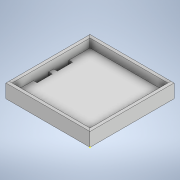
# Autodesk Inventor part: led-compartment
Saved by Autodesk Inventor 2021 (Build 250183000, 183)
## iProperties
Created: 2021-01-17
Part Number: led-compartment
Material: Generic
Document SubType Name: Modeling
Designer: Luke Kamols
Density: 1 g/cm^3
Appearance: Default
Author: Luke Kamols
Autodesk Inventor part; units mm, degrees
ref_plane "YZ Plane" through (0, 0, 0) normal (1, 0, 0) x (0, 1, 0)
ref_plane "XZ Plane" through (0, 0, 0) normal (0, 1, 0) x (-1, 0, 0)
ref_plane "XY Plane" through (0, 0, 0) normal (0, 0, 1) x (1, 0, 0)
sketch "Sketch1" plane through (0, 0, 0) normal (0, 1, 0) x (-1, 0, 0)
  point P0 (0, 0)
sketch "Sketch2" plane through (0, 0, 0) normal (0, 1, 0) x (-1, 0, 0)
  line L0 (0, 0) -> (33.2, 0)
  line L1 (33.2, 0) -> (33.2, -33.2)
  line L2 (33.2, -33.2) -> (0, -33.2)
  line L3 (0, -33.2) -> (0, 0)
  dimension "d0" = 33.2
  dimension "d1" = 33.2
  constraints: 8 end point, 2 parallel, 1 horizontal, 1 perpendicular
  measures "d0" distance of L1.end L2.end
  measures "d1" distance of L0.end L1.end
extrude "Extrusion1" add sketch "Sketch2" along normal blind 2
sketch "Sketch3" plane through (0, 2, 0) normal (0, 1, 0) x (1, 0, 0)
  line L0 (0, 33.2) -> (-33.2, 33.2) projected
  line L1 (-33.2, 33.2) -> (-33.2, 0) projected
  line L2 (-33.2, 0) -> (0, 0) projected
  line L3 (0, 0) -> (0, 33.2) projected
  line L4 (-33.2, 0) -> (0, 0) projected
  line L5 (0, 0) -> (-1.2, 0)
  line L6 (-1.2, 0) -> (-1.2, 1.2)
  line L7 (-1.2, 1.2) -> (-32, 1.2)
  line L8 (-32, 1.2) -> (-32, 32)
  line L9 (-32, 32) -> (-1.2, 32)
  line L10 (-1.2, 32) -> (-1.2, 1.2)
  dimension "d4" = 1.2
  dimension "d5" = 1.2
  dimension "d6" = 30.8
  dimension "d7" = 30.8
  constraints: 12 end point, 2 parallel, 2 perpendicular, 1 horizontal, 1 point on line
  measures "d4" distance of L4.end L5.end
  measures "d5" distance of L5.end L6.end
  measures "d6" distance of L8.end L9.end
  measures "d7" distance of L7.end L8.end
extrude "Extrusion2" add sketch "Sketch3" along normal blind 4
chamfer "Chamfer1" distance 0.6 angle 45 8 edges at (-1.2, 6, -16.6) (-16.6, 6, -32) (-16.6, 6, -33.2) (0, 6, -16.6) (-16.6, 6, 0) (-16.6, 6, -1.2) (-33.2, 6, -16.6) (-32, 6, -16.6)
sketch "Sketch4" plane through (0, 2, 0) normal (0, 1, 0) x (1, 0, 0)
  line L0 (-1.2, 1.2) -> (-1.2, 32) projected
  line L1 (-1.2, 32) -> (-32, 32) projected
  line L2 (-32, 32) -> (-32, 1.2) projected
  line L3 (-32, 1.2) -> (-1.2, 1.2) projected
  line L4 (-1.2, 1.2) -> (-1.2, 32) projected
  line L5 (-1.2, 16.6) -> (-32, 16.6)
  line L6 (-32, 32) -> (-1.2, 32) projected
  line L7 (-16.6, 32) -> (-16.6, 1.2)
  line L8 (-16.6, 16.6) -> (-16.6, 17.6)
  line L9 (-32, 16.6) -> (-32, 17.6)
  line L10 (-32, 1.2) -> (-32, 32) projected
  line L11 (-32, 17.6) -> (-30.5, 17.6)
  line L12 (-30.5, 17.6) -> (-30.5, 23.6)
  line L13 (-30.5, 23.6) -> (-32, 23.6)
  line L14 (-30.5, 16.6) -> (-30.5, 15.6)
  line L15 (-30.5, 15.6) -> (-32, 15.6)
  line L16 (-30.5, 15.6) -> (-30.5, 9.6)
  line L17 (-30.5, 9.6) -> (-32, 9.6)
  line L18 (-1.2, 16.6) -> (-1.2, 17.6)
  line L19 (-1.2, 17.6) -> (-2.7, 17.6)
  line L20 (-2.7, 17.6) -> (-2.7, 23.6)
  line L21 (-2.7, 23.6) -> (-1.2, 23.6)
  line L22 (-1.2, 16.6) -> (-1.2, 15.6)
  line L23 (-1.2, 15.6) -> (-2.7, 15.6)
  line L24 (-2.7, 9.6) -> (-2.7, 15.6)
  line L25 (-2.7, 9.6) -> (-1.2, 9.6)
  point P0 (0, 0)
  dimension "d13" = 1
  dimension "d14" = 1.5
  dimension "d15" = 6
  dimension "d16" = 1
  dimension "d17" = 6
  dimension "d18" = 1
  dimension "d19" = 1.5
  dimension "d20" = 6
  constraints: 38 end point, 10 perpendicular, 10 point on line, 5 midpoint, 2 vertical, 1 horizontal
  measures "d13" distance of L8.start L8.end
  measures "d14" distance of L9.end L11.end
  measures "d15" distance of L11.end L12.end
  measures "d16" distance of L14.start L14.end
  measures "d17" distance of L14.end L16.end
  measures "d18" distance of L5.start L18.end
  measures "d19" distance of L18.end L19.end
  measures "d20" distance of L19.end L20.end
extrude "Extrusion3" cut sketch "Sketch4" against normal blind 4 contours L25 L24 L23 L0 | L2 L15 L16 L17 | L19 L20 L21 L0 | L2 L13 L12 L11
sketch "Sketch5" plane through (0, 0, 0) normal (0, -1, 0) x (1, 0, 0)
  line L0 (-1.2, -17.6) -> (-1.2, -23.6) projected
  line L1 (-1.2, -23.6) -> (-2.7, -23.6) projected
  line L2 (-2.7, -23.6) -> (-2.7, -17.6) projected
  line L3 (-2.7, -17.6) -> (-1.2, -17.6) projected
  line L4 (-32, -23.6) -> (-32, -17.6) projected
  line L5 (-32, -17.6) -> (-30.5, -17.6) projected
  line L6 (-30.5, -17.6) -> (-30.5, -23.6) projected
  line L7 (-30.5, -23.6) -> (-32, -23.6) projected
  line L8 (-1.2, -9.6) -> (-1.2, -15.6) projected
  line L9 (-1.2, -15.6) -> (-2.7, -15.6) projected
  line L10 (-2.7, -15.6) -> (-2.7, -9.6) projected
  line L11 (-2.7, -9.6) -> (-1.2, -9.6) projected
  line L12 (-32, -15.6) -> (-32, -9.6) projected
  line L13 (-32, -9.6) -> (-30.5, -9.6) projected
  line L14 (-30.5, -9.6) -> (-30.5, -15.6) projected
  line L15 (-30.5, -15.6) -> (-32, -15.6) projected
  line L16 (0, -33.2) -> (-33.2, -33.2) projected
  line L17 (0, 0) -> (0, -33.2) projected
  line L18 (-33.2, 0) -> (0, 0) projected
  line L19 (-33.2, -33.2) -> (-33.2, 0) projected
  line L20 (-33.2, 0) -> (0, 0) projected
  line L21 (-16.6, 0) -> (-16.6, -33.2)
  line L22 (0, -33.2) -> (-33.2, -33.2) projected
  line L23 (-16.6, -16.6) -> (-16.6, -1.6)
  line L24 (-1.2, -1.2) -> (-32, -1.2) projected
  line L25 (-16.6, -1.6) -> (-10.1, -1.6)
  line L26 (-10.1, -1.6) -> (-10.1, -31.6)
  line L27 (-10.1, -31.6) -> (-23.1, -31.6)
  line L28 (-23.1, -31.6) -> (-23.1, -1.6)
  line L29 (-23.1, -1.6) -> (-16.6, -1.6)
  line L30 (-10.1, -1.6) -> (-11.1, -1.6)
  line L31 (-11.1, -1.6) -> (-11.1, -2.6)
  line L32 (-11.1, -2.6) -> (-22.1, -2.6)
  line L33 (-22.1, -2.6) -> (-22.1, -30.6)
  line L34 (-22.1, -30.6) -> (-11.1, -30.6)
  line L35 (-11.1, -30.6) -> (-11.1, -2.6)
  dimension "d25" = 6.5
  dimension "d26" = 30
  dimension "d27" = 13
  dimension "d28" = 1
  dimension "d29" = 1
  dimension "d30" = 11
  dimension "d31" = 28
  constraints: 26 end point, 5 perpendicular, 4 parallel, 3 midpoint, 3 point on line, 1 horizontal
  measures "d25" distance of L23.end L25.end
  measures "d26" distance of L25.end L26.end
  measures "d27" distance of L26.end L27.end
  measures "d28" distance of L25.end L30.end
  measures "d29" distance of L30.end L31.end
  measures "d30" distance of L34.end L33.end
  measures "d31" distance of L33.end L32.end
extrude "Extrusion4" cut sketch "Sketch5" against normal blind 1 contours L27 L28 L29 L21 L32 L33 L34 | L21 L34 L35 L31 L25 L26 L27 | L25 L31 L32 L21
chamfer "Chamfer2" distance 0.5 angle 45 8 edges at (-11.1, 1, -16.6) (-16.6, 1, -2.6) (-23.1, 1, -16.6) (-16.6, 1, -1.6) (-22.1, 1, -16.6) (-10.1, 1, -16.6) (-16.6, 1, -30.6) (-16.6, 1, -31.6)
body "Solid1"
